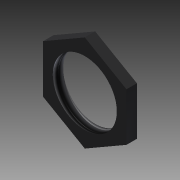
# Autodesk Inventor part: Switch Nut
Saved by Autodesk Inventor 2015 (Build 190159000, 159)
## iProperties
Created: 2016-02-20
Part Number: Switch Nut
Material: Generic
Document SubType Name: Modeling
Designer: 23902
Density: 1 g/cm^3
Appearance: Default
Author: 23902
Autodesk Inventor part; units mm, degrees
ref_plane "YZ Plane" through (0, 0, 0) normal (1, 0, 0) x (0, 1, 0)
ref_plane "XZ Plane" through (0, 0, 0) normal (0, 1, 0) x (-1, 0, 0)
ref_plane "XY Plane" through (0, 0, 0) normal (0, 0, 1) x (1, 0, 0)
sketch "Sketch1" plane through (0, 0, 0) normal (0, 1, 0) x (-1, 0, 0)
  circle A0 centre (0, 0) radius 6.15
  line L0 (0, -9.2376) -> (-8, -4.6188)
  line L1 (-8, -4.6188) -> (-8, 4.6188)
  line L2 (-8, 4.6188) -> (0, 9.2376)
  line L3 (0, 9.2376) -> (8, 4.6188)
  line L4 (8, 4.6188) -> (8, -4.6188)
  line L5 (8, -4.6188) -> (0, -9.2376)
  dimension "d0" = 12.3
  dimension "d1" = 16
  constraints: 12 end point, 2 coincident, 1 centre point, 13 other
  measures "d0" diameter of A0
  measures "d1" distance between parallel lines of L0 L3
extrude "Extrusion1" add sketch "Sketch1" along normal blind 2
thread "Thread1" size "M14x2" class "6H" standard "ANSI Metric M Profile" full length
body "Solid1"
